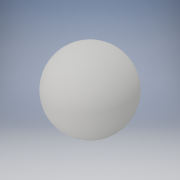
# Autodesk Inventor part: Kugel_Voll
Saved by Autodesk Inventor 2017.3 (Build 213257000, 257)
## iProperties
Part Number: Kugel_Voll
Material: Generisch
Document SubType Name: Modeling
Designer: Enno-LT
Density: 1 g/cm^3
Appearance: Vorgabe
Author: Enno-LT
Autodesk Inventor part; units mm, degrees
ref_plane "YZ Plane" through (0, 0, 0) normal (1, 0, 0) x (0, 1, 0)
ref_plane "XZ Plane" through (0, 0, 0) normal (0, 1, 0) x (-1, 0, 0)
ref_plane "XY Plane" through (0, 0, 0) normal (0, 0, 1) x (1, 0, 0)
sketch "Skizze2" plane through (0, 0, 0) normal (0, 0, 1) x (1, 0, 0)
  line L0 (0, 90) -> (0, 95)
  arc A0 (0, -95) -> (0, 95) centre (0, 0) ccw
  line L1 (0, -95) -> (0, -90)
  arc A1 (0, -90) -> (0, 90) centre (0, 0) ccw
  line L2 (0, 129.0476) -> (0, -140.3376) construction
  dimension "d1" = 5
  dimension "d2" = 5
  dimension "d3" = 190
  constraints: 6 end point, 5 point on line, 4 point on circle, 2 centre point, 2 vertical, 1 coincident
  measures "d1" distance of L0.start L0.end
  measures "d2" distance of L1.start L1.end
  measures "d3" distance of L1.start L0.end
revolve "Umdrehung1" add sketch "Skizze2" angle 360 about axis through (0, 129.0476, 0) along (0, -1, 0)
